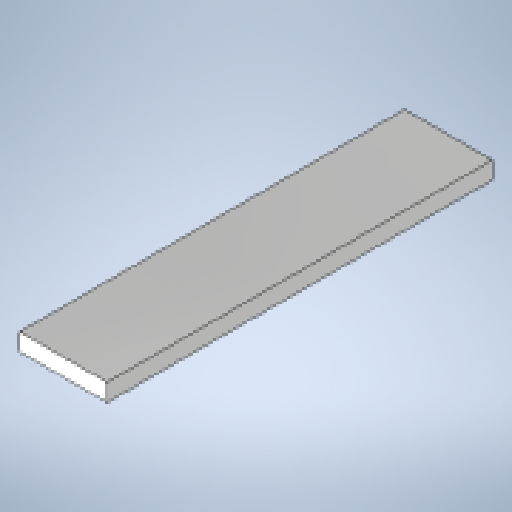
# Autodesk Inventor part: Back Plate
Saved by Autodesk Inventor 2023.2 (Build 272271000, 271)
## iProperties
Created: 2024-03-02
Part Number: Back Plate
Material: UHMW, White
Document SubType Name: Modeling
Designer: Nathan Cai
Mass: 26.4754 g
Surface Area: 110.484 cm^2
Volume: 28.1653 cm^3
Density: 0.94 g/cm^3
Appearance: Smooth - White
Author: Nathan Cai
Autodesk Inventor part; units mm, degrees
ref_plane "YZ Plane" through (0, 0, 0) normal (1, 0, 0) x (0, 1, 0)
ref_plane "XZ Plane" through (0, 0, 0) normal (0, 1, 0) x (-1, 0, 0)
ref_plane "XY Plane" through (0, 0, 0) normal (0, 0, 1) x (1, 0, 0)
sketch "Sketch1" plane through (0, 0, 0) normal (0, 1, 0) x (-1, 0, 0)
  line L0 (-15.875, -69.85) -> (15.875, -69.85)
  line L1 (15.875, -69.85) -> (15.875, 69.85)
  line L2 (15.875, 69.85) -> (-15.875, 69.85)
  line L3 (-15.875, 69.85) -> (-15.875, -69.85)
  line L4 (-15.875, -69.85) -> (15.875, 69.85) construction
  line L5 (15.875, -69.85) -> (-15.875, 69.85) construction
  point P0 (0, 0)
  dimension "d0" = 31.75
  dimension "d1" = 139.7
  constraints: 12 end point, 2 midpoint, 2 parallel, 1 horizontal, 1 perpendicular
  measures "d0" distance of L2.end L1.end
  measures "d1" distance of L1.end L0.end
extrude "Extrusion1" add sketch "Sketch1" along normal blind 6.35
body "Solid1"
